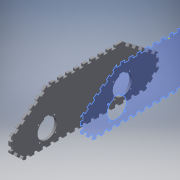
# Autodesk Inventor part: боковина
Saved by Autodesk Inventor 2019 (Build 230136000, 136)
## iProperties
Created: 2022-02-24
Part Number: боковина
Material: Типовые
Document SubType Name: Modeling
Designer: korsh
Density: 1 g/cm^3
Appearance: По умолчанию
Author: korsh
Autodesk Inventor part; units mm, degrees
ref_plane "YZ Plane" through (0, 0, 0) normal (1, 0, 0) x (0, 1, 0)
ref_plane "XZ Plane" through (0, 0, 0) normal (0, 1, 0) x (-1, 0, 0)
ref_plane "XY Plane" through (0, 0, 0) normal (0, 0, 1) x (1, 0, 0)
sketch "Эскиз1" plane through (0, 0, 0) normal (1, 0, 0) x (0, 1, 0)
  circle A0 centre (-36.8789, 121.9871) radius 32.5 projected
  circle A1 centre (-36.8789, 308.3349) radius 32.5 projected
  circle A2 centre (-15.5948, 290.1418) radius 2 projected
  circle A3 centre (-18.6858, 329.619) radius 2 projected
  circle A4 centre (-58.163, 326.528) radius 2 projected
  circle A5 centre (-55.0719, 287.0508) radius 2 projected
  circle A6 centre (-36.8789, 308.3349) radius 23.891 projected
  circle A7 centre (-36.8789, 121.9871) radius 23.891 projected
  circle A8 centre (-18.6858, 143.2712) radius 2 projected
  circle A9 centre (-15.5948, 103.7941) radius 2 projected
  circle A10 centre (-55.0719, 100.703) radius 2 projected
  circle A11 centre (-58.163, 140.1802) radius 2 projected
  arc A12 (-11.5577, 114.2052) -> (-9.5577, 116.2052) centre (-11.5577, 116.2052) ccw projected
  arc A13 (-9.5577, 127.553) -> (-11.5577, 129.553) centre (-11.5577, 127.553) ccw projected
  line L0 (-9.5577, 116.2052) -> (-9.5577, 127.553)
  line L1 (-11.5577, 114.2052) -> (-14.2908, 114.2052)
  line L2 (-11.5577, 129.553) -> (-14.2175, 129.553)
  arc A14 (-60.7699, 308.3349) -> (-36.8789, 284.4439) centre (-36.8789, 308.3349) ccw projected
  arc A15 (-36.8789, 284.4439) -> (-17.3728, 294.5402) centre (-36.8789, 308.3349) ccw projected
  arc A16 (-17.3728, 294.5402) -> (-14.2908, 300.553) centre (-36.8789, 308.3349) ccw projected
  line L3 (-14.2908, 300.553) -> (-11.5577, 300.553) projected
  arc A17 (-11.5577, 300.553) -> (-9.5577, 302.553) centre (-11.5577, 302.553) ccw projected
  line L4 (-9.5577, 302.553) -> (-9.5577, 307.3349) projected
  line L5 (-9.5577, 307.3349) -> (-9.5577, 309.3349) projected
  line L6 (-9.5577, 309.3349) -> (-9.5577, 313.9008) projected
  arc A18 (-9.5577, 313.9008) -> (-11.5577, 315.9008) centre (-11.5577, 313.9008) ccw projected
  line L7 (-11.5577, 315.9008) -> (-14.2175, 315.9008) projected
  arc A19 (-14.2175, 315.9008) -> (-17.111, 321.7517) centre (-36.8789, 308.3349) ccw projected
  arc A20 (-17.111, 321.7517) -> (-36.8789, 332.2259) centre (-36.8789, 308.3349) ccw projected
  arc A21 (-36.8789, 332.2259) -> (-60.7699, 308.3349) centre (-36.8789, 308.3349) ccw projected
  circle A22 centre (-36.8789, 308.3349) radius 32.5 projected
  circle A23 centre (-55.0719, 287.0508) radius 2 projected
  circle A24 centre (-15.5948, 290.1418) radius 2 projected
  circle A25 centre (-18.6858, 329.619) radius 2 projected
  circle A26 centre (-58.163, 326.528) radius 2 projected
  line L8 (-9.5577, 127.553) -> (-9.5577, 116.2052) projected
  line L9 (-11.5577, 114.2052) -> (-14.2908, 114.2052) projected
  line L10 (-14.2175, 129.553) -> (-11.5577, 129.553) projected
  line L11 (-76.5577, 64.2052) -> (-76.5577, 365.9008)
  circle A27 centre (-43.8789, 121.9872) radius 6 projected
  circle A28 centre (-43.8789, 308.335) radius 6 projected
  line L12 (-46.4674, 32.0244) -> (-46.4674, 398.2977) construction
  line L13 (-76.5577, 64.2052) -> (-46.4674, 32.0244)
  line L14 (-76.5577, 365.9008) -> (-46.4674, 398.2977)
  line L15 (-46.4674, 32.0244) -> (-11.4674, 32.0244)
  line L16 (-46.4674, 398.2977) -> (-11.4674, 398.2977)
  line L17 (-43.8789, 121.9872) -> (56.1211, 121.9872) construction
  line L18 (-43.8789, 308.335) -> (56.1211, 308.335) construction
  line L19 (-11.4674, 32.0244) -> (56.1211, 121.9872)
  line L20 (-11.4674, 398.2977) -> (56.1211, 308.335)
  line L21 (56.1211, 121.9872) -> (56.1211, 308.335)
  point P0 (0, 0)
  dimension "d0" = 67
  dimension "d1" = 50
  dimension "d2" = 67
  dimension "d3" = 50
  dimension "d4" = 90
  dimension "d6" = 90
  dimension "d7" = 34.3212
  dimension "d8" = 35
  dimension "d9" = 35
  dimension "d10" = 100
  constraints: 28 end point, 4 horizontal, 4 vertical, 2 point on circle, 1 parallel, 1 perpendicular
  measures "d0" distance between parallel lines of L11 L0
  measures "d1" distance from line of L11.start L1
  measures "d2" distance from line of L5.end L11
  measures "d3" distance from line of L7 L11.end
  measures "d4" distance of L12.start L17.start
  measures "d6" distance of L12.end L18.start
  measures "d7" distance from line of L17.start L0
  measures "d8" distance of L12.start L15.end
  measures "d9" distance of L12.end L16.end
  measures "d10" distance of L17.start L17.end
extrude "Выдавливание1" add sketch "Эскиз1" along normal blind 6 contours A0 | A1 | L11 L14 L16 L20 L21 L19 L15 L13
sketch "Эскиз2" plane through (0, 0, 0) normal (-1, 0, 0) x (0, 0, 1)
  point P0 (0, 0)
sketch "Эскиз3" plane through (6, 0, 0) normal (1, 0, 0) x (0, 0, -1)
  line L0 (-121.9872, 56.1211) -> (-308.335, 56.1211) projected
  line L1 (-308.335, 56.1211) -> (-298.335, 56.1211)
  line L2 (-298.335, 56.1211) -> (-298.335, 50.1211)
  line L3 (-298.335, 50.1211) -> (-308.335, 50.1211)
  line L4 (-308.335, 50.1211) -> (-308.335, 56.1211)
  line L5 (-288.335, 56.1211) -> (-278.335, 56.1211)
  line L6 (-278.335, 56.1211) -> (-278.335, 50.1211)
  line L7 (-278.335, 50.1211) -> (-288.335, 50.1211)
  line L8 (-288.335, 50.1211) -> (-288.335, 56.1211)
  line L9 (-268.335, 56.1211) -> (-258.335, 56.1211)
  line L10 (-258.335, 56.1211) -> (-258.335, 50.1211)
  line L11 (-258.335, 50.1211) -> (-268.335, 50.1211)
  line L12 (-268.335, 50.1211) -> (-268.335, 56.1211)
  line L13 (-248.335, 56.1211) -> (-238.335, 56.1211)
  line L14 (-238.335, 56.1211) -> (-238.335, 50.1211)
  line L15 (-238.335, 50.1211) -> (-248.335, 50.1211)
  line L16 (-248.335, 50.1211) -> (-248.335, 56.1211)
  line L17 (-228.335, 56.1211) -> (-218.335, 56.1211)
  line L18 (-218.335, 56.1211) -> (-218.335, 50.1211)
  line L19 (-218.335, 50.1211) -> (-228.335, 50.1211)
  line L20 (-228.335, 50.1211) -> (-228.335, 56.1211)
  line L21 (-208.335, 56.1211) -> (-198.335, 56.1211)
  line L22 (-198.335, 56.1211) -> (-198.335, 50.1211)
  line L23 (-198.335, 50.1211) -> (-208.335, 50.1211)
  line L24 (-208.335, 50.1211) -> (-208.335, 56.1211)
  line L25 (-188.335, 56.1211) -> (-178.335, 56.1211)
  line L26 (-178.335, 56.1211) -> (-178.335, 50.1211)
  line L27 (-178.335, 50.1211) -> (-188.335, 50.1211)
  line L28 (-188.335, 50.1211) -> (-188.335, 56.1211)
  line L29 (-168.335, 56.1211) -> (-158.335, 56.1211)
  line L30 (-158.335, 56.1211) -> (-158.335, 50.1211)
  line L31 (-158.335, 50.1211) -> (-168.335, 50.1211)
  line L32 (-168.335, 50.1211) -> (-168.335, 56.1211)
  line L33 (-148.335, 56.1211) -> (-138.335, 56.1211)
  line L34 (-138.335, 56.1211) -> (-138.335, 50.1211)
  line L35 (-138.335, 50.1211) -> (-148.335, 50.1211)
  line L36 (-148.335, 50.1211) -> (-148.335, 56.1211)
  line L37 (-365.9008, -76.5577) -> (-64.2052, -76.5577) projected
  line L38 (-359.9008, -76.5577) -> (-349.9008, -76.5577)
  line L39 (-349.9008, -76.5577) -> (-349.9008, -70.5577)
  line L40 (-349.9008, -70.5577) -> (-359.9008, -70.5577)
  line L41 (-359.9008, -70.5577) -> (-359.9008, -76.5577)
  line L42 (-386.6987, -10.2578) -> (-378.7037, -4.2512)
  line L43 (-378.7037, -4.2512) -> (-382.3077, 0.5458)
  line L44 (-382.3077, 0.5458) -> (-390.3027, -5.4608)
  line L45 (-390.3027, -5.4608) -> (-386.6987, -10.2578)
  line L46 (-386.6987, -10.2578) -> (-382.3077, 0.5458) construction
  line L47 (-378.7037, -4.2512) -> (-390.3027, -5.4608) construction
  line L48 (-308.335, 56.1211) -> (-398.2977, -11.4674) projected
  line L49 (-362.7136, 7.762) -> (-366.3176, 12.5591)
  line L50 (-370.7087, 1.7554) -> (-362.7136, 7.762)
  line L51 (-370.7087, 1.7554) -> (-366.3176, 12.5591) construction
  line L52 (-366.3176, 12.5591) -> (-374.3126, 6.5524)
  line L53 (-362.7136, 7.762) -> (-374.3126, 6.5524) construction
  line L54 (-374.3126, 6.5524) -> (-370.7087, 1.7554)
  line L55 (-346.7236, 19.7753) -> (-350.3276, 24.5723)
  line L56 (-354.7186, 13.7687) -> (-346.7236, 19.7753)
  line L57 (-354.7186, 13.7687) -> (-350.3276, 24.5723) construction
  line L58 (-350.3276, 24.5723) -> (-358.3226, 18.5657)
  line L59 (-346.7236, 19.7753) -> (-358.3226, 18.5657) construction
  line L60 (-358.3226, 18.5657) -> (-354.7186, 13.7687)
  line L61 (-330.7335, 31.7885) -> (-334.3375, 36.5856)
  line L62 (-338.7286, 25.7819) -> (-330.7335, 31.7885)
  line L63 (-338.7286, 25.7819) -> (-334.3375, 36.5856) construction
  line L64 (-334.3375, 36.5856) -> (-342.3325, 30.5789)
  line L65 (-330.7335, 31.7885) -> (-342.3325, 30.5789) construction
  line L66 (-342.3325, 30.5789) -> (-338.7286, 25.7819)
  line L67 (-314.7435, 43.8018) -> (-318.3474, 48.5988)
  line L68 (-322.7385, 37.7952) -> (-314.7435, 43.8018)
  line L69 (-322.7385, 37.7952) -> (-318.3474, 48.5988) construction
  line L70 (-318.3474, 48.5988) -> (-326.3425, 42.5922)
  line L71 (-314.7435, 43.8018) -> (-326.3425, 42.5922) construction
  line L72 (-326.3425, 42.5922) -> (-322.7385, 37.7952)
  line L73 (-32.0244, -11.4674) -> (-121.9872, 56.1211) projected
  line L74 (-40.0195, -5.4608) -> (-43.6234, -10.2578)
  line L75 (-43.6234, -10.2578) -> (-51.6185, -4.2512)
  line L76 (-51.6185, -4.2512) -> (-48.0084, 0.5412)
  line L77 (-48.0084, 0.5412) -> (-40.0195, -5.4608)
  line L78 (-67.6085, 7.7621) -> (-63.9984, 12.5545)
  line L79 (-59.6135, 1.7554) -> (-67.6085, 7.7621)
  line L80 (-63.9984, 12.5545) -> (-56.0095, 6.5524)
  line L81 (-56.0095, 6.5524) -> (-59.6135, 1.7554)
  line L82 (-83.5986, 19.7753) -> (-79.9885, 24.5677)
  line L83 (-75.6035, 13.7687) -> (-83.5986, 19.7753)
  line L84 (-79.9885, 24.5677) -> (-71.9996, 18.5657)
  line L85 (-71.9996, 18.5657) -> (-75.6035, 13.7687)
  line L86 (-99.5886, 31.7885) -> (-95.9785, 36.581)
  line L87 (-91.5936, 25.7819) -> (-99.5886, 31.7885)
  line L88 (-95.9785, 36.581) -> (-87.9896, 30.5789)
  line L89 (-87.9896, 30.5789) -> (-91.5936, 25.7819)
  line L90 (-115.5787, 43.8018) -> (-111.9686, 48.5942)
  line L91 (-107.5837, 37.7952) -> (-115.5787, 43.8018)
  line L92 (-111.9686, 48.5942) -> (-103.9797, 42.5922)
  line L93 (-103.9797, 42.5922) -> (-107.5837, 37.7952)
  line L94 (-339.9008, -76.5577) -> (-329.9008, -76.5577)
  line L95 (-329.9008, -76.5577) -> (-329.9008, -70.5577)
  line L96 (-329.9008, -70.5577) -> (-339.9008, -70.5577)
  line L97 (-339.9008, -70.5577) -> (-339.9008, -76.5577)
  line L98 (-319.9008, -76.5577) -> (-309.9008, -76.5577)
  line L99 (-309.9008, -76.5577) -> (-309.9008, -70.5577)
  line L100 (-309.9008, -70.5577) -> (-319.9008, -70.5577)
  line L101 (-319.9008, -70.5577) -> (-319.9008, -76.5577)
  line L102 (-299.9008, -76.5577) -> (-289.9008, -76.5577)
  line L103 (-289.9008, -76.5577) -> (-289.9008, -70.5577)
  line L104 (-289.9008, -70.5577) -> (-299.9008, -70.5577)
  line L105 (-299.9008, -70.5577) -> (-299.9008, -76.5577)
  line L106 (-279.9008, -76.5577) -> (-269.9008, -76.5577)
  line L107 (-269.9008, -76.5577) -> (-269.9008, -70.5577)
  line L108 (-269.9008, -70.5577) -> (-279.9008, -70.5577)
  line L109 (-279.9008, -70.5577) -> (-279.9008, -76.5577)
  line L110 (-259.9008, -76.5577) -> (-249.9008, -76.5577)
  line L111 (-249.9008, -76.5577) -> (-249.9008, -70.5577)
  line L112 (-249.9008, -70.5577) -> (-259.9008, -70.5577)
  line L113 (-259.9008, -70.5577) -> (-259.9008, -76.5577)
  line L114 (-239.9008, -76.5577) -> (-229.9008, -76.5577)
  line L115 (-229.9008, -76.5577) -> (-229.9008, -70.5577)
  line L116 (-229.9008, -70.5577) -> (-239.9008, -70.5577)
  line L117 (-239.9008, -70.5577) -> (-239.9008, -76.5577)
  line L118 (-219.9008, -76.5577) -> (-209.9008, -76.5577)
  line L119 (-209.9008, -76.5577) -> (-209.9008, -70.5577)
  line L120 (-209.9008, -70.5577) -> (-219.9008, -70.5577)
  line L121 (-219.9008, -70.5577) -> (-219.9008, -76.5577)
  line L122 (-199.9008, -76.5577) -> (-189.9008, -76.5577)
  line L123 (-189.9008, -76.5577) -> (-189.9008, -70.5577)
  line L124 (-189.9008, -70.5577) -> (-199.9008, -70.5577)
  line L125 (-199.9008, -70.5577) -> (-199.9008, -76.5577)
  line L126 (-179.9008, -76.5577) -> (-169.9008, -76.5577)
  line L127 (-169.9008, -76.5577) -> (-169.9008, -70.5577)
  line L128 (-169.9008, -70.5577) -> (-179.9008, -70.5577)
  line L129 (-179.9008, -70.5577) -> (-179.9008, -76.5577)
  line L130 (-159.9008, -76.5577) -> (-149.9008, -76.5577)
  line L131 (-149.9008, -76.5577) -> (-149.9008, -70.5577)
  line L132 (-149.9008, -70.5577) -> (-159.9008, -70.5577)
  line L133 (-159.9008, -70.5577) -> (-159.9008, -76.5577)
  line L134 (-139.9008, -76.5577) -> (-129.9008, -76.5577)
  line L135 (-129.9008, -76.5577) -> (-129.9008, -70.5577)
  line L136 (-129.9008, -70.5577) -> (-139.9008, -70.5577)
  line L137 (-139.9008, -70.5577) -> (-139.9008, -76.5577)
  line L138 (-119.9008, -76.5577) -> (-109.9008, -76.5577)
  line L139 (-109.9008, -76.5577) -> (-109.9008, -70.5577)
  line L140 (-109.9008, -70.5577) -> (-119.9008, -70.5577)
  line L141 (-119.9008, -70.5577) -> (-119.9008, -76.5577)
  line L142 (-99.9008, -76.5577) -> (-89.9008, -76.5577)
  line L143 (-89.9008, -76.5577) -> (-89.9008, -70.5577)
  line L144 (-89.9008, -70.5577) -> (-99.9008, -70.5577)
  line L145 (-99.9008, -70.5577) -> (-99.9008, -76.5577)
  line L146 (-79.9008, -76.5577) -> (-69.9008, -76.5577)
  line L147 (-69.9008, -76.5577) -> (-69.9008, -70.5577)
  line L148 (-69.9008, -70.5577) -> (-79.9008, -70.5577)
  line L149 (-79.9008, -70.5577) -> (-79.9008, -76.5577)
  line L150 (-398.2977, -11.4674) -> (-392.2977, -11.4674)
  line L151 (-392.2977, -11.4674) -> (-392.2977, -21.4674)
  line L152 (-392.2977, -21.4674) -> (-398.2977, -21.4674)
  line L153 (-398.2977, -21.4674) -> (-398.2977, -11.4674)
  line L154 (-392.2977, -41.4674) -> (-398.2977, -41.4674)
  line L155 (-398.2977, -41.4674) -> (-398.2977, -31.4674)
  line L156 (-392.2977, -31.4674) -> (-392.2977, -41.4674)
  line L157 (-398.2977, -31.4674) -> (-392.2977, -31.4674)
  line L158 (-32.0244, -46.4674) -> (-32.0244, -11.4674) projected
  line L159 (-32.0244, -11.4674) -> (-38.0244, -11.4674)
  line L160 (-38.0244, -11.4674) -> (-38.0244, -21.4674)
  line L161 (-38.0244, -21.4674) -> (-32.0244, -21.4674)
  line L162 (-32.0244, -21.4674) -> (-32.0244, -11.4674)
  line L163 (-32.0244, -31.4674) -> (-38.0244, -31.4674)
  line L164 (-38.0244, -31.4674) -> (-38.0244, -41.4674)
  line L165 (-38.0244, -41.4674) -> (-32.0244, -41.4674)
  line L166 (-32.0244, -41.4674) -> (-32.0244, -31.4674)
  line L167 (-398.2977, -46.4674) -> (-365.9008, -76.5577) projected
  line L168 (-64.2052, -76.5577) -> (-32.0244, -46.4674) projected
  line L169 (-392.2977, -52.0402) -> (-388.2145, -47.644)
  line L170 (-388.2145, -47.644) -> (-380.8874, -54.4494)
  line L171 (-380.8874, -54.4494) -> (-384.9706, -58.8456)
  line L172 (-392.2977, -52.0402) -> (-384.9706, -58.8456)
  line L173 (-373.5603, -61.2548) -> (-366.2332, -68.0602)
  line L174 (-377.6435, -65.6511) -> (-370.3164, -72.4565)
  line L175 (-366.2332, -68.0602) -> (-370.3164, -72.4565)
  line L176 (-377.6435, -65.6511) -> (-373.5603, -61.2548)
  line L177 (-38.4413, -52.4674) -> (-42.5392, -48.0848)
  line L178 (-42.5392, -48.0848) -> (-49.8435, -54.9147)
  line L179 (-49.8435, -54.9147) -> (-45.7456, -59.2973)
  line L180 (-38.4413, -52.4674) -> (-45.7456, -59.2973)
  line L181 (-53.0499, -66.1271) -> (-57.1478, -61.7445)
  line L182 (-57.1478, -61.7445) -> (-64.4522, -68.5743)
  line L183 (-64.4522, -68.5743) -> (-60.3543, -72.9569)
  line L184 (-53.0499, -66.1271) -> (-60.3543, -72.9569)
  point P0 (-384.5032, -4.856)
  point P1 (-368.5131, 7.1572)
  point P2 (-352.5231, 19.1705)
  point P3 (-336.533, 31.1837)
  point P4 (-320.543, 43.197)
  point P5 (-52.6331, -55.1271)
  dimension "d13" = 10
  dimension "d14" = 6
  dimension "d17" = 20
  dimension "d32" = 6
  dimension "d33" = 10
  dimension "d34" = 6
  dimension "d35" = 10
  dimension "d36" = 6
  dimension "d39" = 20
  dimension "d44" = 10
  dimension "d49" = 6
  dimension "d50" = 10
  dimension "d51" = 6
  dimension "d52" = 10
  dimension "d55" = 20
  dimension "d62" = 20
  dimension "d67" = 6
  dimension "d68" = 10
  dimension "d71" = 20
  dimension "d76" = 6
  dimension "d77" = 10
  dimension "d80" = 20
  dimension "d85" = 6
  dimension "d86" = 10
  dimension "d87" = 90
  dimension "d88" = 90
  dimension "d91" = 20
  dimension "d97" = 90
  dimension "d99" = 6
  dimension "d100" = 10
  dimension "d103" = 20
  dimension "d109" = 6
  dimension "d110" = 6
  constraints: 356 end point, 11 parallel, 10 midpoint, 8 perpendicular, 7 point on line, 6 horizontal, 4 collinear, 2 vertical, 288 other
  measures "d13" distance of L2.end L3.end
  measures "d14" distance of L1.end L2.end
  measures "d17" distance of L2.end L6.end
  measures "d32" distance of L38.end L39.end
  measures "d33" distance of L39.end L40.end
  measures "d34" distance from line of L37.start L41
  measures "d35" distance of L43.end L44.end
  measures "d36" distance of L44.end L42.start
  measures "d39" distance of L42.end L49.start
  measures "d44" distance from line of L45 L48.end
  measures "d49" distance of L74.start L74.end
  measures "d50" distance of L74.end L75.end
  measures "d51" distance of L75.end L76.end
  measures "d52" distance from line of L73.start L74
  measures "d55" distance of L75.end L78.start
  measures "d62" distance of L38.start L94.start
  measures "d67" distance of L151.end L152.end
  measures "d68" distance of L150.end L151.end
  measures "d71" distance of L152.end L154.end
  measures "d76" distance of L161.end L160.end
  measures "d77" distance of L160.end L159.end
  measures "d80" distance of L159.end L163.end
  measures "d85" distance of L169.start L169.end
  measures "d86" distance of L169.end L170.end
  measures "d87" angle of L167 L169
  measures "d88" angle of L170 L169
  measures "d91" distance of L169.end L173.start
  measures "d97" angle of L168 L177
  measures "d99" distance of L177.start L177.end
  measures "d100" distance of L177.end L178.end
  measures "d103" distance of L164.end point (-52.633, -55.127)
  measures "d109" horizontal distance of L169.start L167.start
  measures "d110" vertical distance of L158.start L177.start
extrude "Выдавливание2" cut sketch "Эскиз3" against normal blind 6
equation "\"d6\" = d4"
equation "\"d52\" = d44"
